Autodesk Inventor part; units mm, degrees
(part 4 of 6)
sketch "Sketch55" plane through (0, 0, 10) normal (0, 0, 1) x (1, 0, 0)
  line L0 (103.1549, -6.3815) -> (106.5137, -3.0228) projected
  line L1 (103.1549, -6.3815) -> (104.357, -7.5836) projected
  line L2 (104.357, -7.5836) -> (100.1144, -11.8263) projected
  line L3 (100.1144, -11.8263) -> (83.8509, -28.0897) projected
  line L4 (83.8509, -28.0897) -> (80.3154, -31.6252) projected
  line L5 (80.3154, -31.6252) -> (71.5473, -22.8571) projected
  line L6 (71.5473, -22.8571) -> (75.0828, -19.3216) projected
  line L7 (75.0828, -19.3216) -> (91.3463, -3.0581) projected
  line L8 (91.3463, -3.0581) -> (95.5889, 1.1845) projected
  line L9 (95.5889, 1.1845) -> (96.791, -0.0176) projected
  line L10 (100.1497, 3.3412) -> (96.791, -0.0176) projected
  line L11 (106.5137, -3.0228) -> (100.1497, 3.3412) projected
  line L12 (4.5, 17.5) -> (4.5, 22.25) projected
  line L13 (4.5, 17.5) -> (6.2, 17.5) projected
  line L14 (6.2, 17.5) -> (6.2, 11.5) projected
  line L15 (6.2, 11.5) -> (6.2, -11.5) projected
  line L16 (6.2, -11.5) -> (6.2, -16.5) projected
  line L17 (6.2, -16.5) -> (-6.2, -16.5) projected
  line L18 (-6.2, -16.5) -> (-6.2, -11.5) projected
  line L19 (-6.2, -11.5) -> (-6.2, 11.5) projected
  line L20 (-6.2, 11.5) -> (-6.2, 17.5) projected
  line L21 (-6.2, 17.5) -> (-4.5, 17.5) projected
  line L22 (-4.5, 22.25) -> (-4.5, 17.5) projected
  line L23 (4.5, 22.25) -> (-4.5, 22.25) projected
  line L24 (-103.1549, -136.2186) -> (-106.5137, -139.5774) projected
  line L25 (-103.1549, -136.2186) -> (-104.357, -135.0165) projected
  line L26 (-104.357, -135.0165) -> (-100.1144, -130.7739) projected
  line L27 (-100.1144, -130.7739) -> (-83.8509, -114.5104) projected
  line L28 (-83.8509, -114.5104) -> (-80.3154, -110.9749) projected
  line L29 (-80.3154, -110.9749) -> (-71.5473, -119.743) projected
  line L30 (-71.5473, -119.743) -> (-75.0828, -123.2786) projected
  line L31 (-75.0828, -123.2786) -> (-91.3463, -139.542) projected
  line L32 (-91.3463, -139.542) -> (-95.5889, -143.7847) projected
  line L33 (-95.5889, -143.7847) -> (-96.791, -142.5826) projected
  line L34 (-100.1497, -145.9413) -> (-96.791, -142.5826) projected
  line L35 (-106.5137, -139.5774) -> (-100.1497, -145.9413) projected
  line L36 (-96.791, -0.0176) -> (-100.1497, 3.3412) projected
  line L37 (-96.791, -0.0176) -> (-95.5889, 1.1845) projected
  line L38 (-95.5889, 1.1845) -> (-91.3463, -3.0581) projected
  line L39 (-91.3463, -3.0581) -> (-75.0828, -19.3216) projected
  line L40 (-75.0828, -19.3216) -> (-71.5473, -22.8571) projected
  line L41 (-71.5473, -22.8571) -> (-80.3154, -31.6252) projected
  line L42 (-80.3154, -31.6252) -> (-83.8509, -28.0897) projected
  line L43 (-83.8509, -28.0897) -> (-100.1144, -11.8263) projected
  line L44 (-100.1144, -11.8263) -> (-104.357, -7.5836) projected
  line L45 (-104.357, -7.5836) -> (-103.1549, -6.3815) projected
  line L46 (-106.5137, -3.0228) -> (-103.1549, -6.3815) projected
  line L47 (-100.1497, 3.3412) -> (-106.5137, -3.0228) projected
  line L48 (-4.5, -160.1002) -> (-4.5, -164.8502) projected
  line L49 (-4.5, -160.1002) -> (-6.2, -160.1002) projected
  line L50 (-6.2, -160.1002) -> (-6.2, -154.1002) projected
  line L51 (-6.2, -154.1002) -> (-6.2, -131.1002) projected
  line L52 (-6.2, -131.1002) -> (-6.2, -126.1002) projected
  line L53 (-6.2, -126.1002) -> (6.2, -126.1002) projected
  line L54 (6.2, -126.1002) -> (6.2, -131.1002) projected
  line L55 (6.2, -131.1002) -> (6.2, -154.1002) projected
  line L56 (6.2, -154.1002) -> (6.2, -160.1002) projected
  line L57 (6.2, -160.1002) -> (4.5, -160.1002) projected
  line L58 (4.5, -164.8502) -> (4.5, -160.1002) projected
  line L59 (-4.5, -164.8502) -> (4.5, -164.8502) projected
  line L60 (96.791, -142.5826) -> (100.1497, -145.9413) projected
  line L61 (96.791, -142.5826) -> (95.5889, -143.7847) projected
  line L62 (95.5889, -143.7847) -> (91.3463, -139.542) projected
  line L63 (91.3463, -139.542) -> (75.0828, -123.2786) projected
  line L64 (75.0828, -123.2786) -> (71.5473, -119.743) projected
  line L65 (71.5473, -119.743) -> (80.3154, -110.9749) projected
  line L66 (80.3154, -110.9749) -> (83.8509, -114.5104) projected
  line L67 (83.8509, -114.5104) -> (100.1144, -130.7739) projected
  line L68 (100.1144, -130.7739) -> (104.357, -135.0165) projected
  line L69 (104.357, -135.0165) -> (103.1549, -136.2186) projected
  line L70 (106.5137, -139.5774) -> (103.1549, -136.2186) projected
  line L71 (100.1497, -145.9413) -> (106.5137, -139.5774) projected
  circle A0 centre (27.1, -49.4001) radius 1.5 projected
  circle A1 centre (-27.1, -49.4001) radius 1.5 projected
  circle A2 centre (27.1, -93.2001) radius 1.5 projected
  circle A3 centre (-27.1, -93.2001) radius 1.5 projected
  line L72 (4.575, -111.1002) -> (4.575, -104.5252) projected
  line L73 (4.575, -104.5252) -> (6.575, -104.5252) projected
  line L74 (6.575, -104.5252) -> (6.575, -111.1002) projected
  line L75 (6.575, -111.1002) -> (4.575, -111.1002) projected
  line L76 (62.0897, -34.6128) -> (57.4405, -39.262) projected
  line L77 (57.4405, -39.262) -> (56.0263, -37.8478) projected
  line L78 (56.0263, -37.8478) -> (60.6755, -33.1986) projected
  line L79 (60.6755, -33.1986) -> (62.0897, -34.6128) projected
  line L80 (-62.0897, -34.6128) -> (-57.4405, -39.262) projected
  line L81 (-62.0897, -34.6128) -> (-60.6755, -33.1986) projected
  line L82 (-60.6755, -33.1986) -> (-56.0263, -37.8478) projected
  line L83 (-56.0263, -37.8478) -> (-57.4405, -39.262) projected
  line L84 (-62.0897, -107.9874) -> (-57.4405, -103.3382) projected
  line L85 (-57.4405, -103.3382) -> (-56.0263, -104.7524) projected
  line L86 (-56.0263, -104.7524) -> (-60.6755, -109.4016) projected
  line L87 (-60.6755, -109.4016) -> (-62.0897, -107.9874) projected
  line L88 (68.5597, -101.5174) -> (63.9105, -96.8681) projected
  line L89 (63.9105, -96.8681) -> (65.3247, -95.4539) projected
  line L90 (65.3247, -95.4539) -> (69.974, -100.1031) projected
  line L91 (69.974, -100.1031) -> (68.5597, -101.5174) projected
  line L92 (84.2822, -48.8001) -> (88.2822, -48.8001) projected
  line L93 (88.2822, -48.8001) -> (94.3529, -27.4901) projected
  line L94 (94.3529, -27.4901) -> (106.8333, -15.0097) projected
  arc A4 (106.8333, -15.0097) -> (88.1629, 3.6608) centre (97.4981, -5.6744) ccw projected
  line L95 (88.1629, 3.6608) -> (75.6824, -8.8196) projected
  line L96 (75.6824, -8.8196) -> (57.202, -21.3001) projected
  line L97 (57.202, -21.3001) -> (38.202, -31.3001) projected
  line L98 (38.202, -31.3001) -> (19.202, -21.3001) projected
  line L99 (19.202, -21.3001) -> (13.202, -3.65) projected
  line L100 (13.202, -3.65) -> (13.202, 14) projected
  arc A5 (13.202, 14) -> (-13.202, 14) centre (0, 14) ccw projected
  line L101 (-13.202, 14) -> (-13.202, -3.65) projected
  line L102 (-13.202, -3.65) -> (-19.202, -21.3001) projected
  line L103 (-19.202, -21.3001) -> (-38.202, -31.3001) projected
  line L104 (-38.202, -31.3001) -> (-57.202, -21.3001) projected
  line L105 (-57.202, -21.3001) -> (-75.6824, -8.8196) projected
  line L106 (-75.6824, -8.8196) -> (-88.1629, 3.6608) projected
  arc A6 (-88.1629, 3.6608) -> (-106.8333, -15.0097) centre (-97.4981, -5.6744) ccw projected
  line L107 (-106.8333, -15.0097) -> (-94.3529, -27.4901) projected
  line L108 (-94.3529, -27.4901) -> (-76.3482, -71.3001) projected
  line L109 (-76.3482, -71.3001) -> (-94.3529, -115.1101) projected
  line L110 (-94.3529, -115.1101) -> (-106.8333, -127.5905) projected
  arc A7 (-106.8333, -127.5905) -> (-88.1629, -146.2609) centre (-97.4981, -136.9257) ccw projected
  line L111 (-88.1629, -146.2609) -> (-75.6824, -133.7805) projected
  line L112 (-75.6824, -133.7805) -> (-57.202, -121.3001) projected
  line L113 (-57.202, -121.3001) -> (-38.202, -111.3001) projected
  line L114 (-38.202, -111.3001) -> (-19.202, -121.3001) projected
  line L115 (-19.202, -121.3001) -> (-13.202, -138.9501) projected
  line L116 (-13.202, -138.9501) -> (-13.202, -156.6002) projected
  arc A8 (-13.202, -156.6002) -> (13.202, -156.6002) centre (0, -156.6002) ccw projected
  line L117 (13.202, -156.6002) -> (13.202, -138.9501) projected
  line L118 (13.202, -138.9501) -> (19.202, -121.3001) projected
  line L119 (19.202, -121.3001) -> (38.202, -111.3001) projected
  line L120 (38.202, -111.3001) -> (57.202, -121.3001) projected
  line L121 (57.202, -121.3001) -> (75.6824, -133.7805) projected
  line L122 (75.6824, -133.7805) -> (88.1629, -146.2609) projected
  arc A9 (88.1629, -146.2609) -> (106.8333, -127.5905) centre (97.4981, -136.9257) ccw projected
  line L123 (106.8333, -127.5905) -> (94.3529, -115.1101) projected
  line L124 (94.3529, -115.1101) -> (88.2822, -93.8001) projected
  line L125 (88.2822, -93.8001) -> (84.2822, -93.8001) projected
  line L126 (84.2822, -48.8001) -> (84.2822, -93.8001) projected
  line L127 (-54.1, -54.2001) -> (44.1, -54.2001) projected
  arc A10 (44.1, -64.2001) -> (44.1, -54.2001) centre (44.1, -59.2001) ccw projected
  line L128 (44.1, -64.2001) -> (44.1, -78.4001) projected
  arc A11 (44.1, -88.4001) -> (44.1, -78.4001) centre (44.1, -83.4001) ccw projected
  line L129 (44.1, -88.4001) -> (-54.1, -88.4001) projected
  line L130 (-54.1, -54.2001) -> (-54.1, -88.4001) projected
  line L131 (-4.575, -38.075) -> (-4.575, -31.5) projected
  line L132 (-4.575, -38.075) -> (-6.575, -38.075) projected
  line L133 (-6.575, -38.075) -> (-6.575, -31.5) projected
  line L134 (-6.575, -31.5) -> (-4.575, -31.5) projected
  line L135 (-4.575, -111.1002) -> (-6.575, -111.1002) projected
  line L136 (-6.575, -111.1002) -> (-6.575, -104.5252) projected
  line L137 (-6.575, -104.5252) -> (-4.575, -104.5252) projected
  line L138 (-4.575, -111.1002) -> (-4.575, -104.5252) projected
  line L139 (4.575, -31.5) -> (6.575, -31.5) projected
  line L140 (6.575, -31.5) -> (6.575, -38.075) projected
  line L141 (6.575, -38.075) -> (4.575, -38.075) projected
  line L142 (4.575, -38.075) -> (4.575, -31.5) projected
  line L143 (68.5597, -41.0828) -> (69.974, -42.497) projected
  line L144 (69.974, -42.497) -> (65.3247, -47.1462) projected
  line L145 (65.3247, -47.1462) -> (63.9105, -45.732) projected
  line L146 (68.5597, -41.0828) -> (63.9105, -45.732) projected
  line L147 (62.0897, -107.9874) -> (60.6755, -109.4016) projected
  line L148 (60.6755, -109.4016) -> (56.0263, -104.7524) projected
  line L149 (56.0263, -104.7524) -> (57.4405, -103.3382) projected
  line L150 (62.0897, -107.9874) -> (57.4405, -103.3382) projected
  line L151 (-68.5597, -101.5174) -> (-69.974, -100.1031) projected
  line L152 (-69.974, -100.1031) -> (-65.3247, -95.4539) projected
  line L153 (-65.3247, -95.4539) -> (-63.9105, -96.8681) projected
  line L154 (-68.5597, -101.5174) -> (-63.9105, -96.8681) projected
  line L155 (-63.9105, -45.732) -> (-65.3247, -47.1462) projected
  line L156 (-65.3247, -47.1462) -> (-69.974, -42.497) projected
  line L157 (-69.974, -42.497) -> (-68.5597, -41.0828) projected
  line L158 (-68.5597, -41.0828) -> (-63.9105, -45.732) projected
  line L159 (106.8333, -15.0097) -> (94.3529, -27.4901) projected
  line L160 (75.6824, -8.8196) -> (94.3529, -27.4901)
  line L161 (94.3529, -115.1101) -> (88.2822, -93.8001) projected
  line L162 (94.3529, -115.1101) -> (75.6824, -133.7805)
  line L163 (13.202, -138.9501) -> (-13.202, -138.9501)
  line L164 (-57.202, -121.3001) -> (-75.6824, -133.7805) projected
  line L165 (-75.6824, -133.7805) -> (-94.3529, -115.1101)
  line L166 (-94.3529, -27.4901) -> (-75.6824, -8.8196)
  line L167 (-19.202, -21.3001) -> (-13.202, -3.65) projected
  line L168 (-13.202, -3.65) -> (13.202, -3.65)
  line L169 (6.2, 11.5) -> (6.2, -11.5) projected
  line L170 (94.3529, -27.4901) -> (88.2822, -48.8001) projected
  line L171 (84.2822, -48.8001) -> (88.2822, -48.8001) projected
  line L172 (94.3529, -27.4901) -> (88.2822, -48.8001)
  line L173 (88.2822, -48.8001) -> (84.4352, -47.7042)
  line L174 (84.4352, -47.7042) -> (90.5059, -26.3942)
  line L175 (90.5059, -26.3942) -> (94.3529, -27.4901)
  line L176 (84.4352, -47.7042) -> (84.2822, -48.8001)
  line L177 (90.5059, -26.3942) -> (91.8815, -25.0187)
  line L178 (88.2822, -93.8001) -> (94.3529, -115.1101)
  line L179 (94.3529, -115.1101) -> (90.5059, -116.206)
  line L180 (90.5059, -116.206) -> (84.4352, -94.896)
  line L181 (84.4352, -94.896) -> (88.2822, -93.8001)
  line L182 (84.2822, -93.8001) -> (84.4352, -94.896)
  line L183 (90.5059, -116.206) -> (91.8815, -117.5815)
  line L184 (75.6824, -8.8196) -> (88.1629, 3.6608) projected
  line L185 (57.202, -21.3001) -> (75.6824, -8.8196) projected
  line L186 (75.6824, -8.8196) -> (57.202, -21.3001)
  line L187 (57.202, -21.3001) -> (59.4406, -24.615)
  line L188 (59.4406, -24.615) -> (77.9211, -12.1345)
  line L189 (77.9211, -12.1345) -> (75.6824, -8.8196)
  line L190 (77.9211, -12.1345) -> (78.4592, -11.5964)
  line L191 (38.202, -31.3001) -> (57.202, -21.3001) projected
  line L192 (38.202, -31.3001) -> (57.202, -21.3001)
  line L193 (57.202, -21.3001) -> (59.065, -24.8397)
  line L194 (59.065, -24.8397) -> (40.065, -34.8397)
  line L195 (40.065, -34.8397) -> (38.202, -31.3001)
  line L196 (59.065, -24.8397) -> (59.4406, -24.615)
  line L197 (19.202, -21.3001) -> (38.202, -31.3001)
  line L198 (38.202, -31.3001) -> (36.339, -34.8397)
  line L199 (36.339, -34.8397) -> (17.339, -24.8397)
  line L200 (17.339, -24.8397) -> (19.202, -21.3001)
  line L201 (36.339, -34.8397) -> (40.065, -34.8397)
  line L202 (13.202, 14) -> (13.202, -3.65) projected
  line L203 (13.202, -3.65) -> (19.202, -21.3001)
  line L204 (19.202, -21.3001) -> (15.4148, -22.5875)
  line L205 (15.4148, -22.5875) -> (9.4148, -4.9375)
  line L206 (9.4148, -4.9375) -> (13.202, -3.65)
  line L207 (15.4148, -22.5875) -> (17.339, -24.8397)
  line L208 (9.4148, -4.9375) -> (9.4148, -3.65)
  line L209 (-13.202, -3.65) -> (-19.202, -21.3001)
  line L210 (-19.202, -21.3001) -> (-15.4148, -22.5875)
  line L211 (-15.4148, -22.5875) -> (-9.4148, -4.9375)
  line L212 (-9.4148, -4.9375) -> (-13.202, -3.65)
  line L213 (-9.4148, -4.9375) -> (-9.4148, -3.65)
  line L214 (-38.202, -31.3001) -> (-19.202, -21.3001) projected
  line L215 (-19.202, -21.3001) -> (-38.202, -31.3001)
  line L216 (-38.202, -31.3001) -> (-36.339, -34.8397)
  line L217 (-36.339, -34.8397) -> (-17.339, -24.8397)
  line L218 (-17.339, -24.8397) -> (-19.202, -21.3001)
  line L219 (-15.4148, -22.5875) -> (-17.339, -24.8397)
  line L220 (-75.6824, -8.8196) -> (-57.202, -21.3001) projected
  line L221 (-38.202, -31.3001) -> (-57.202, -21.3001)
  line L222 (-57.202, -21.3001) -> (-59.065, -24.8397)
  line L223 (-59.065, -24.8397) -> (-40.065, -34.8397)
  line L224 (-40.065, -34.8397) -> (-38.202, -31.3001)
  line L225 (-40.065, -34.8397) -> (-36.339, -34.8397)
  line L226 (-75.6824, -8.8196) -> (-57.202, -21.3001)
  line L227 (-57.202, -21.3001) -> (-59.4406, -24.615)
  line L228 (-59.4406, -24.615) -> (-77.9211, -12.1345)
  line L229 (-77.9211, -12.1345) -> (-75.6824, -8.8196)
  line L230 (-59.4406, -24.615) -> (-59.065, -24.8397)
  line L231 (-77.9211, -12.1345) -> (-78.4592, -11.5964)
  line L232 (-94.3529, -27.4901) -> (-76.3482, -71.3001)
  line L233 (-76.3482, -71.3001) -> (-72.6485, -69.7796)
  line L234 (-72.6485, -69.7796) -> (-90.6531, -25.9696)
  line L235 (-90.6531, -25.9696) -> (-94.3529, -27.4901)
  line L236 (-90.6531, -25.9696) -> (-91.7428, -24.88)
  line L237 (-94.3529, -115.1101) -> (-76.3482, -71.3001) projected
  line L238 (-76.3482, -71.3001) -> (-94.3529, -115.1101)
  line L239 (-94.3529, -115.1101) -> (-90.6531, -116.6306)
  line L240 (-90.6531, -116.6306) -> (-72.6485, -72.8206)
  line L241 (-72.6485, -72.8206) -> (-76.3482, -71.3001)
  line L242 (-72.6485, -69.7796) -> (-72.6485, -72.8206)
  line L243 (-90.6531, -116.6306) -> (-91.7428, -117.7202)
  line L244 (-75.6824, -133.7805) -> (-57.202, -121.3001)
  line L245 (-57.202, -121.3001) -> (-59.4406, -117.9852)
  line L246 (-59.4406, -117.9852) -> (-77.9211, -130.4656)
  line L247 (-77.9211, -130.4656) -> (-75.6824, -133.7805)
  line L248 (-77.9211, -130.4656) -> (-78.4592, -131.0037)
  line L249 (-57.202, -121.3001) -> (-38.202, -111.3001)
  line L250 (-38.202, -111.3001) -> (-40.065, -107.7604)
  line L251 (-40.065, -107.7604) -> (-59.065, -117.7604)
  line L252 (-59.065, -117.7604) -> (-57.202, -121.3001)
  line L253 (-59.065, -117.7604) -> (-59.4406, -117.9852)
  line L254 (-19.202, -121.3001) -> (-38.202, -111.3001) projected
  line L255 (-19.202, -121.3001) -> (-38.202, -111.3001)
  line L256 (-38.202, -111.3001) -> (-36.339, -107.7604)
  line L257 (-36.339, -107.7604) -> (-17.339, -117.7604)
  line L258 (-17.339, -117.7604) -> (-19.202, -121.3001)
  line L259 (-40.065, -107.7604) -> (-36.339, -107.7604)
  line L260 (-13.202, -138.9501) -> (-19.202, -121.3001) projected
  line L261 (-19.202, -121.3001) -> (-13.202, -138.9501)
  line L262 (-13.202, -138.9501) -> (-9.4148, -137.6627)
  line L263 (-9.4148, -137.6627) -> (-15.4148, -120.0127)
  line L264 (-15.4148, -120.0127) -> (-19.202, -121.3001)
  line L265 (-17.339, -117.7604) -> (-15.4148, -120.0127)
  line L266 (-9.4148, -137.6627) -> (-9.4148, -138.9501)
  line L267 (13.202, -138.9501) -> (19.202, -121.3001)
  line L268 (19.202, -121.3001) -> (15.4148, -120.0127)
  line L269 (15.4148, -120.0127) -> (9.4148, -137.6627)
  line L270 (9.4148, -137.6627) -> (13.202, -138.9501)
  line L271 (9.4148, -137.6627) -> (9.4148, -138.9501)
  line L272 (57.202, -121.3001) -> (38.202, -111.3001) projected
  line L273 (19.202, -121.3001) -> (38.202, -111.3001)
  line L274 (38.202, -111.3001) -> (36.339, -107.7604)
  line L275 (36.339, -107.7604) -> (17.339, -117.7604)
  line L276 (17.339, -117.7604) -> (19.202, -121.3001)
  line L277 (17.339, -117.7604) -> (15.4148, -120.0127)
  line L278 (75.6824, -133.7805) -> (57.202, -121.3001) projected
  line L279 (57.202, -121.3001) -> (38.202, -111.3001)
  line L280 (38.202, -111.3001) -> (40.065, -107.7604)
  line L281 (40.065, -107.7604) -> (59.065, -117.7604)
  line L282 (59.065, -117.7604) -> (57.202, -121.3001)
  line L283 (36.339, -107.7604) -> (40.065, -107.7604)
  line L284 (57.202, -121.3001) -> (75.6824, -133.7805)
  line L285 (75.6824, -133.7805) -> (77.9211, -130.4656)
  line L286 (77.9211, -130.4656) -> (59.4406, -117.9852)
  line L287 (59.4406, -117.9852) -> (57.202, -121.3001)
  line L288 (59.065, -117.7604) -> (59.4406, -117.9852)
  line L289 (77.9211, -130.4656) -> (78.4592, -131.0037)
  line L290 (-72.6485, -71.3001) -> (-67.6485, -71.3001)
  line L291 (-67.6485, -71.3001) -> (-67.6485, -56.3001)
  line L292 (-67.6485, -56.3001) -> (-78.1882, -56.3001)
  line L293 (-67.6485, -71.3001) -> (-67.6485, -86.3001)
  line L294 (-67.6485, -71.3001) -> (-52.6485, -71.3001) construction
  line L295 (-67.6485, -86.3001) -> (-78.1882, -86.3001)
  line L296 (84.4352, -94.896) -> (86.627, -102.5899)
  line L297 (86.627, -102.5899) -> (78.9331, -104.7817)
  line L298 (78.9331, -104.7817) -> (76.7413, -97.0878)
  line L299 (76.7413, -97.0878) -> (84.4352, -94.896)
  line L300 (84.4352, -47.7042) -> (86.627, -40.0103)
  line L301 (86.627, -40.0103) -> (78.9331, -37.8185)
  line L302 (78.9331, -37.8185) -> (76.7413, -45.5124)
  line L303 (76.7413, -45.5124) -> (84.4352, -47.7042)
  point P0 (0, 0)
  dimension "d720" = 4
  dimension "d722" = 4
  dimension "d724" = 4
  dimension "d725" = 4
  dimension "d726" = 4
  dimension "d728" = 4
  dimension "d729" = 4
  dimension "d731" = 4
  dimension "d732" = 4
  dimension "d733" = 4
  dimension "d734" = 4
  dimension "d736" = 4
  dimension "d737" = 4
  dimension "d738" = 4
  dimension "d739" = 4
  dimension "d740" = 4
  dimension "d741" = 4
  dimension "d742" = 4
  dimension "d743" = 4
  dimension "d744" = 4
  dimension "d745" = 4
  dimension "d746" = 5
  dimension "d747" = 15
  dimension "d748" = 15
  dimension "d749" = 90
  dimension "d750" = 8
  dimension "d751" = 8
  dimension "d752" = 8
  dimension "d753" = 8
  constraints: 254 end point, 56 equal length, 41 perpendicular, 16 point on line, 3 horizontal, 1 midpoint
  measures "d720" distance of L92.start L92.end
  measures "d722" distance of L92.end L173.end
  measures "d724" distance of L180.end L124.end
  measures "d725" distance of L96.end L187.end
  measures "d726" distance of L194.end L97.end
  measures "d728" distance of L97.end L198.end
  measures "d729" distance of L98.end L204.end
  measures "d731" distance of L102.end L210.end
  measures "d732" distance of L103.end L216.end
  measures "d733" distance of L104.end L222.end
  measures "d734" distance of L104.end L227.end
  measures "d736" distance of L108.end L233.end
  measures "d737" distance of L109.end L239.end
  measures "d738" distance of L112.end L245.end
  measures "d739" distance of L113.end L250.end
  measures "d740" distance of L113.end L256.end
  measures "d741" distance of L263.end L114.end
  measures "d742" distance of L118.end L268.end
  measures "d743" distance of L119.end L274.end
  measures "d744" distance of L119.end L280.end
  measures "d745" distance of L121.end L285.end
  measures "d746" distance of L290.start L290.end
  measures "d747" distance of L290.end L291.end
  measures "d748" distance of L290.end L293.end
  measures "d749" angle of L293 L294
  measures "d750" distance of L180.end L296.end
  measures "d751" distance of L296.end L297.end
  measures "d752" distance of L302.end L173.end
  measures "d753" distance of L300.end L173.end
extrude "Extrusion55" add sketch "Sketch55" along normal up to surface (25 mm away) contours L160 L175 L177 | L190 L189 L160 | L93 L173 L174 L175 | L189 L188 L187 L96 | L92 L176 L173 | L174 L303 L302 L301 | L193 L194 L195 L97 | L187 L196 L193 | L198 L199 L200 L98 | L195 L201 L198 | L125 L181 L182 | L204 L205 L206 L99 | L200 L207 L204 | L124 L179 L180 L181 | L180 L297 L298 L299 | L206 L208 L168 | L162 L183 L179 | L212 L211 L210 L102 | L168 L213 L212 | L285 L289 L162 | L121 L287 L286 L285 | L218 L217 L216 L103 | L210 L219 L218 | L120 L280 L281 L282 | L282 L288 L287 | L224 L223 L222 L104 | L216 L225 L224 | L119 L276 L275 L274 | L274 L283 L280 | L227 L228 L229 L105 | L222 L230 L227 | L118 L270 L269 L268 | L268 L277 L276 | L229 L231 L166 | L163 L271 L270 | L235 L234 L233 L108 | L166 L236 L235 | L262 L266 L163 | L115 L264 L263 L262 | L241 L240 L239 L109 | L233 L242 L241 | L114 L256 L257 L258 | L258 L265 L264 | L239 L243 L165 | L234 L292 L291 L290 L242 | L242 L290 L293 L295 L240 | L113 L252 L251 L250 | L250 L259 L256 | L112 L247 L246 L245 | L245 L253 L252 | L165 L248 L247
sketch "Sketch56" plane through (-78.1882, -86.3001, 35) normal (0, 0, 1) x (1, 0, 0)
  line L0 (0, 0) -> (-12.465, -30.3305) projected
  line L1 (10.5397, 0) -> (0, 0) projected
  line L2 (10.5397, 30) -> (10.5397, 0) projected
  line L3 (0, 30) -> (10.5397, 30) projected
  line L4 (-12.465, 60.3305) -> (0, 30) projected
  line L5 (-13.5546, 61.4201) -> (-12.465, 60.3305) projected
  line L6 (-16.1647, 58.81) -> (-13.5546, 61.4201) projected
  line L7 (1.84, 15) -> (-16.1647, 58.81) projected
  line L8 (-16.1647, -28.81) -> (1.84, 15) projected
  line L9 (-13.5546, -31.4201) -> (-16.1647, -28.81) projected
  line L10 (-12.465, -30.3305) -> (-13.5546, -31.4201) projected
  line L11 (68.7733, 81.3626) -> (62.7733, 63.7126) projected
  line L12 (68.7733, 82.65) -> (68.7733, 81.3626) projected
  line L13 (64.9862, 82.65) -> (68.7733, 82.65) projected
  line L14 (58.9862, 65) -> (64.9862, 82.65) projected
  line L15 (39.9862, 55) -> (58.9862, 65) projected
  line L16 (20.9862, 65) -> (39.9862, 55) projected
  line L17 (2.5057, 77.4804) -> (20.9862, 65) projected
  line L18 (-0.271, 74.7037) -> (2.5057, 77.4804) projected
  line L19 (0.2671, 74.1656) -> (-0.271, 74.7037) projected
  line L20 (18.7475, 61.6851) -> (0.2671, 74.1656) projected
  line L21 (19.1232, 61.4603) -> (18.7475, 61.6851) projected
  line L22 (38.1232, 51.4603) -> (19.1232, 61.4603) projected
  line L23 (41.8491, 51.4603) -> (38.1232, 51.4603) projected
  line L24 (60.8491, 61.4603) -> (41.8491, 51.4603) projected
  line L25 (62.7733, 63.7126) -> (60.8491, 61.4603) projected
  line L26 (95.5272, 61.4603) -> (93.603, 63.7126) projected
  line L27 (114.5272, 51.4603) -> (95.5272, 61.4603) projected
  line L28 (118.2531, 51.4603) -> (114.5272, 51.4603) projected
  line L29 (137.2531, 61.4603) -> (118.2531, 51.4603) projected
  line L30 (137.6288, 61.6851) -> (137.2531, 61.4603) projected
  line L31 (156.1092, 74.1656) -> (137.6288, 61.6851) projected
  line L32 (156.6474, 74.7037) -> (156.1092, 74.1656) projected
  line L33 (153.8706, 77.4804) -> (156.6474, 74.7037) projected
  line L34 (135.3902, 65) -> (153.8706, 77.4804) projected
  line L35 (116.3902, 55) -> (135.3902, 65) projected
  line L36 (97.3902, 65) -> (116.3902, 55) projected
  line L37 (91.3902, 82.65) -> (97.3902, 65) projected
  line L38 (87.603, 82.65) -> (91.3902, 82.65) projected
  line L39 (87.603, 81.3626) -> (87.603, 82.65) projected
  line L40 (93.603, 63.7126) -> (87.603, 81.3626) projected
  line L41 (162.4703, 37.5) -> (162.4703, -7.5) projected
  line L42 (162.6234, -8.5959) -> (162.4703, -7.5) projected
  line L43 (154.9295, -10.7877) -> (162.6234, -8.5959) projected
  line L44 (157.1213, -18.4816) -> (154.9295, -10.7877) projected
  line L45 (164.8152, -16.2898) -> (157.1213, -18.4816) projected
  line L46 (168.6941, -29.9059) -> (164.8152, -16.2898) projected
  line L47 (170.0696, -31.2814) -> (168.6941, -29.9059) projected
  line L48 (172.541, -28.81) -> (170.0696, -31.2814) projected
  line L49 (166.4703, -7.5) -> (172.541, -28.81) projected
  line L50 (166.4703, 37.5) -> (166.4703, -7.5) projected
  line L51 (172.541, 58.81) -> (166.4703, 37.5) projected
  line L52 (170.0696, 61.2814) -> (172.541, 58.81) projected
  line L53 (168.6941, 59.9059) -> (170.0696, 61.2814) projected
  line L54 (164.8152, 46.2898) -> (168.6941, 59.9059) projected
  line L55 (157.1213, 48.4816) -> (164.8152, 46.2898) projected
  line L56 (154.9295, 40.7877) -> (157.1213, 48.4816) projected
  line L57 (162.6234, 38.5959) -> (154.9295, 40.7877) projected
  line L58 (162.4703, 37.5) -> (162.6234, 38.5959) projected
  line L59 (87.603, -51.3626) -> (93.603, -33.7126) projected
  line L60 (87.603, -52.65) -> (87.603, -51.3626) projected
  line L61 (91.3902, -52.65) -> (87.603, -52.65) projected
  line L62 (97.3902, -35) -> (91.3902, -52.65) projected
  line L63 (116.3902, -25) -> (97.3902, -35) projected
  line L64 (135.3902, -35) -> (116.3902, -25) projected
  line L65 (153.8706, -47.4804) -> (135.3902, -35) projected
  line L66 (156.6474, -44.7037) -> (153.8706, -47.4804) projected
  line L67 (156.1092, -44.1656) -> (156.6474, -44.7037) projected
  line L68 (137.6288, -31.6851) -> (156.1092, -44.1656) projected
  line L69 (137.2531, -31.4603) -> (137.6288, -31.6851) projected
  line L70 (118.2531, -21.4603) -> (137.2531, -31.4603) projected
  line L71 (114.5272, -21.4603) -> (118.2531, -21.4603) projected
  line L72 (95.5272, -31.4603) -> (114.5272, -21.4603) projected
  line L73 (93.603, -33.7126) -> (95.5272, -31.4603) projected
  line L74 (39.9862, -25) -> (20.9862, -35) projected
  line L75 (58.9862, -35) -> (39.9862, -25) projected
  line L76 (64.9862, -52.65) -> (58.9862, -35) projected
  line L77 (68.7733, -52.65) -> (64.9862, -52.65) projected
  line L78 (68.7733, -51.3626) -> (68.7733, -52.65) projected
  line L79 (62.7733, -33.7126) -> (68.7733, -51.3626) projected
  line L80 (60.8491, -31.4603) -> (62.7733, -33.7126) projected
  line L81 (41.8491, -21.4603) -> (60.8491, -31.4603) projected
  line L82 (38.1232, -21.4603) -> (41.8491, -21.4603) projected
  line L83 (19.1232, -31.4603) -> (38.1232, -21.4603) projected
  line L84 (18.7475, -31.6851) -> (19.1232, -31.4603) projected
  line L85 (0.2671, -44.1656) -> (18.7475, -31.6851) projected
  line L86 (20.9862, -35) -> (2.5057, -47.4804) projected
  line L87 (-0.271, -44.7037) -> (0.2671, -44.1656) projected
  line L88 (2.5057, -47.4804) -> (-0.271, -44.7037) projected
  point P0 (78.1882, 86.3001)
extrude "Extrusion56" add sketch "Sketch56" along normal blind 20
ref_plane "Work Plane2" through (94.3529, -27.4901, 10) normal (1, 0, 0) x (0, 0, 1)
sketch "Sketch58" plane through (94.3529, -27.4901, 10) normal (1, 0, 0) x (0, 0, 1)
  line L0 (0, -23.8401) -> (45, -23.8401) projected
  line L1 (0, 111.46) -> (45, 111.46) projected
  line L2 (45, -23.8401) -> (45, -22.5526) projected
  arc A0 (45, -23.8401) -> (45, 111.46) centre (-121.8037, 43.81) ccw
  line L3 (45, -23.8401) -> (45, 111.46)
  line L4 (45, 106.2904) -> (45, 93.81) projected
  point P0 (-10, -27.4901)
  dimension "d758" = 180
  constraints: 2 end point, 2 point on circle, 1 centre point, 1 collinear
  measures "d758" radius of A0
extrude "Extrusion57" add sketch "Sketch58" against normal up to surface (188.7058 mm away)
sketch "Sketch61" plane through (94.3529, -27.4901, 55) normal (0, 0, -1) x (-1, 0, 0)
  line L0 (6.0707, -66.31) -> (0, -87.62) projected
  line L1 (0, -87.62) -> (-12.4804, -100.1004) projected
  arc A0 (-12.4804, -100.1004) -> (6.19, -118.7709) centre (-3.1452, -109.4356) ccw projected
  line L2 (6.19, -118.7709) -> (18.6704, -106.2904) projected
  line L3 (18.6704, -106.2904) -> (37.1509, -93.81) projected
  line L4 (37.1509, -93.81) -> (56.1509, -83.81) projected
  line L5 (56.1509, -83.81) -> (75.1509, -93.81) projected
  line L6 (75.1509, -93.81) -> (81.1509, -111.46) projected
  line L7 (81.1509, -111.46) -> (81.1509, -129.1101) projected
  arc A1 (81.1509, -129.1101) -> (107.5549, -129.1101) centre (94.3529, -129.1101) ccw projected
  line L8 (107.5549, -129.1101) -> (107.5549, -111.46) projected
  line L9 (107.5549, -111.46) -> (113.5549, -93.81) projected
  line L10 (113.5549, -93.81) -> (132.5549, -83.81) projected
  line L11 (132.5549, -83.81) -> (151.5549, -93.81) projected
  line L12 (151.5549, -93.81) -> (170.0353, -106.2904) projected
  line L13 (170.0353, -106.2904) -> (182.5158, -118.7709) projected
  arc A2 (182.5158, -118.7709) -> (201.1862, -100.1004) centre (191.851, -109.4356) ccw projected
  line L14 (201.1862, -100.1004) -> (188.7058, -87.62) projected
  line L15 (188.7058, -87.62) -> (170.7011, -43.81) projected
  line L16 (170.7011, -43.81) -> (188.7058, 0) projected
  line L17 (188.7058, 0) -> (201.1862, 12.4804) projected
  arc A3 (201.1862, 12.4804) -> (182.5158, 31.1509) centre (191.851, 21.8157) ccw projected
  line L18 (182.5158, 31.1509) -> (170.0353, 18.6704) projected
  line L19 (170.0353, 18.6704) -> (151.5549, 6.19) projected
  line L20 (151.5549, 6.19) -> (132.5549, -3.81) projected
  line L21 (132.5549, -3.81) -> (113.5549, 6.19) projected
  line L22 (113.5549, 6.19) -> (107.5549, 23.8401) projected
  line L23 (107.5549, 23.8401) -> (107.5549, 41.4901) projected
  arc A4 (107.5549, 41.4901) -> (81.1509, 41.4901) centre (94.3529, 41.4901) ccw projected
  line L24 (81.1509, 41.4901) -> (81.1509, 23.8401) projected
  line L25 (81.1509, 23.8401) -> (75.1509, 6.19) projected
  line L26 (75.1509, 6.19) -> (56.1509, -3.81) projected
  line L27 (56.1509, -3.81) -> (37.1509, 6.19) projected
  line L28 (37.1509, 6.19) -> (18.6704, 18.6704) projected
  line L29 (18.6704, 18.6704) -> (6.19, 31.1509) projected
  arc A5 (6.19, 31.1509) -> (-12.4804, 12.4804) centre (-3.1452, 21.8157) ccw projected
  line L30 (-12.4804, 12.4804) -> (0, 0) projected
  line L31 (0, 0) -> (6.0707, -21.31) projected
  line L32 (6.0707, -66.31) -> (6.0707, -21.31) projected
  line L33 (65.4631, -18.81) -> (69.0427, -18.81) projected
  line L34 (69.0427, -18.81) -> (70.8325, -21.91) projected
  line L35 (70.8325, -21.91) -> (69.0427, -25.01) projected
  line L36 (69.0427, -25.01) -> (65.4631, -25.01) projected
  line L37 (65.4631, -25.01) -> (63.6733, -21.91) projected
  line L38 (63.6733, -21.91) -> (65.4631, -18.81) projected
  line L39 (117.8733, -21.91) -> (119.6631, -18.81) projected
  line L40 (119.6631, -18.81) -> (123.2427, -18.81) projected
  line L41 (123.2427, -18.81) -> (125.0325, -21.91) projected
  line L42 (125.0325, -21.91) -> (123.2427, -25.01) projected
  line L43 (123.2427, -25.01) -> (119.6631, -25.01) projected
  line L44 (119.6631, -25.01) -> (117.8733, -21.91) projected
  line L45 (69.0427, -62.61) -> (70.8325, -65.71) projected
  line L46 (70.8325, -65.71) -> (69.0427, -68.81) projected
  line L47 (69.0427, -68.81) -> (65.4631, -68.81) projected
  line L48 (65.4631, -68.81) -> (63.6733, -65.71) projected
  line L49 (63.6733, -65.71) -> (65.4631, -62.61) projected
  line L50 (65.4631, -62.61) -> (69.0427, -62.61) projected
  line L51 (119.6631, -68.81) -> (117.8733, -65.71) projected
  line L52 (117.8733, -65.71) -> (119.6631, -62.61) projected
  line L53 (119.6631, -62.61) -> (123.2427, -62.61) projected
  line L54 (123.2427, -62.61) -> (125.0325, -65.71) projected
  line L55 (125.0325, -65.71) -> (123.2427, -68.81) projected
  line L56 (123.2427, -68.81) -> (119.6631, -68.81) projected
  line L57 (91.2313, -99.3917) -> (94.3313, -97.6019) projected
  line L58 (94.3313, -97.6019) -> (97.4313, -99.3917) projected
  line L59 (97.4313, -99.3917) -> (97.4313, -102.9713) projected
  line L60 (97.4313, -102.9713) -> (94.3313, -104.7611) projected
  line L61 (94.3313, -104.7611) -> (91.2313, -102.9713) projected
  line L62 (91.2313, -102.9713) -> (91.2313, -99.3917) projected
  line L63 (91.1005, 13.4938) -> (92.7276, 16.3077) projected
  line L64 (92.7276, 16.3077) -> (95.9781, 16.3055) projected
  line L65 (95.9781, 16.3055) -> (97.6015, 13.4894) projected
  line L66 (97.6015, 13.4894) -> (95.9743, 10.6755) projected
  line L67 (95.9743, 10.6755) -> (92.7238, 10.6777) projected
  line L68 (92.7238, 10.6777) -> (91.1005, 13.4938) projected
  line L69 (17.4084, -93.3427) -> (13.8197, -92.2431) projected
  line L70 (13.8197, -92.2431) -> (12.9777, -88.5855) projected
  line L71 (12.9777, -88.5855) -> (15.7243, -86.0274) projected
  line L72 (15.7243, -86.0274) -> (19.313, -87.127) projected
  line L73 (19.313, -87.127) -> (20.155, -90.7847) projected
  line L74 (20.155, -90.7847) -> (17.4084, -93.3427) projected
  line L75 (168.4107, -90.7107) -> (169.2997, -87.0641) projected
  line L76 (169.2997, -87.0641) -> (172.9022, -86.0107) projected
  line L77 (172.9022, -86.0107) -> (175.6157, -88.6039) projected
  line L78 (175.6157, -88.6039) -> (174.7267, -92.2504) projected
  line L79 (174.7267, -92.2504) -> (171.1242, -93.3038) projected
  line L80 (171.1242, -93.3038) -> (168.4107, -90.7107) projected
  line L81 (175.6861, 0.9694) -> (172.9726, -1.6238) projected
  line L82 (172.9726, -1.6238) -> (169.3701, -0.5704) projected
  line L83 (169.3701, -0.5704) -> (168.4811, 3.0762) projected
  line L84 (168.4811, 3.0762) -> (171.1946, 5.6693) projected
  line L85 (171.1946, 5.6693) -> (174.7971, 4.6159) projected
  line L86 (174.7971, 4.6159) -> (175.6861, 0.9694) projected
  line L87 (17.4412, 5.6455) -> (20.1879, 3.0874) projected
  line L88 (20.1879, 3.0874) -> (19.3458, -0.5703) projected
  line L89 (19.3458, -0.5703) -> (15.7571, -1.6699) projected
  line L90 (15.7571, -1.6699) -> (13.0105, 0.8882) projected
  line L91 (13.0105, 0.8882) -> (13.8526, 4.5459) projected
  line L92 (13.8526, 4.5459) -> (17.4412, 5.6455) projected
  circle A6 centre (2.8652, 15.8053) radius 5 projected
  circle A7 centre (94.3529, -120.6101) radius 5 projected
  circle A8 centre (185.8406, 15.8053) radius 5 projected
  circle A9 centre (185.8406, -103.4252) radius 5 projected
  circle A10 centre (2.8652, -103.4252) radius 5 projected
  circle A11 centre (94.3529, 32.9901) radius 5 projected
  line L93 (58.0139, -7.3497) -> (77.0139, 2.6503) projected
  line L94 (54.2879, -7.3497) -> (58.0139, -7.3497) projected
  line L95 (35.2879, 2.6503) -> (54.2879, -7.3497) projected
  line L96 (77.0139, 2.6503) -> (78.938, 4.9026) projected
  line L97 (78.938, 4.9026) -> (84.938, 22.5526) projected
  line L98 (84.938, 22.5526) -> (84.938, 23.8401) projected
  line L99 (84.938, 23.8401) -> (81.1509, 23.8401) projected
  line L100 (18.6704, 18.6704) -> (15.8937, 15.8937) projected
  line L101 (15.8937, 15.8937) -> (16.4318, 15.3556) projected
  line L102 (16.4318, 15.3556) -> (34.9122, 2.8751) projected
  line L103 (158.2634, -18.2419) -> (159.6776, -19.6562) projected
  line L104 (159.6776, -19.6562) -> (164.3268, -15.0069) projected
  line L105 (164.3268, -15.0069) -> (162.9126, -13.5927) projected
  line L106 (162.9126, -13.5927) -> (158.2634, -18.2419) projected
  line L107 (162.9126, -74.0273) -> (164.3268, -72.613) projected
  line L108 (164.3268, -72.613) -> (159.6776, -67.9638) projected
  line L109 (159.6776, -67.9638) -> (158.2634, -69.378) projected
  line L110 (162.9126, -74.0273) -> (158.2634, -69.378) projected
  line L111 (32.2632, -80.4973) -> (33.6774, -81.9115) projected
  line L112 (33.6774, -81.9115) -> (38.3266, -77.2623) projected
  line L113 (38.3266, -77.2623) -> (36.9124, -75.8481) projected
  line L114 (32.2632, -80.4973) -> (36.9124, -75.8481) projected
  line L115 (25.7931, -13.5927) -> (24.3789, -15.0069) projected
  line L116 (24.3789, -15.0069) -> (29.0281, -19.6562) projected
  line L117 (29.0281, -19.6562) -> (30.4424, -18.2419) projected
  line L118 (25.7931, -13.5927) -> (30.4424, -18.2419) projected
  line L119 (89.7779, -4.0099) -> (87.7779, -4.0099) projected
  line L120 (87.7779, -4.0099) -> (87.7779, -10.5849) projected
  line L121 (87.7779, -10.5849) -> (89.7779, -10.5849) projected
  line L122 (89.7779, -10.5849) -> (89.7779, -4.0099) projected
  line L123 (98.9279, -83.6101) -> (100.9279, -83.6101) projected
  line L124 (100.9279, -83.6101) -> (100.9279, -77.0351) projected
  line L125 (100.9279, -77.0351) -> (98.9279, -77.0351) projected
  line L126 (98.9279, -83.6101) -> (98.9279, -77.0351) projected
  line L127 (98.9279, -10.5849) -> (98.9279, -4.0099) projected
  line L128 (98.9279, -10.5849) -> (100.9279, -10.5849) projected
  line L129 (100.9279, -10.5849) -> (100.9279, -4.0099) projected
  line L130 (100.9279, -4.0099) -> (98.9279, -4.0099) projected
  line L131 (148.4529, -26.71) -> (50.2529, -26.71) projected
  arc A12 (50.2529, -26.71) -> (50.2529, -36.71) centre (50.2529, -31.71) ccw projected
  line L132 (50.2529, -36.71) -> (50.2529, -50.91) projected
  arc A13 (50.2529, -50.91) -> (50.2529, -60.91) centre (50.2529, -55.91) ccw projected
  line L133 (50.2529, -60.91) -> (148.4529, -60.91) projected
  line L134 (148.4529, -26.71) -> (148.4529, -60.91) projected
  line L135 (25.7931, -74.0273) -> (30.4424, -69.378) projected
  line L136 (30.4424, -69.378) -> (29.0281, -67.9638) projected
  line L137 (29.0281, -67.9638) -> (24.3789, -72.613) projected
  line L138 (24.3789, -72.613) -> (25.7931, -74.0273) projected
  line L139 (156.4426, -80.4973) -> (151.7934, -75.8481) projected
  line L140 (151.7934, -75.8481) -> (150.3792, -77.2623) projected
  line L141 (150.3792, -77.2623) -> (155.0284, -81.9115) projected
  line L142 (155.0284, -81.9115) -> (156.4426, -80.4973) projected
  line L143 (156.4426, -7.1227) -> (151.7934, -11.7719) projected
  line L144 (156.4426, -7.1227) -> (155.0284, -5.7085) projected
  line L145 (155.0284, -5.7085) -> (150.3792, -10.3577) projected
  line L146 (150.3792, -10.3577) -> (151.7934, -11.7719) projected
  line L147 (32.2632, -7.1227) -> (36.9124, -11.7719) projected
  line L148 (36.9124, -11.7719) -> (38.3266, -10.3577) projected
  line L149 (38.3266, -10.3577) -> (33.6774, -5.7085) projected
  line L150 (33.6774, -5.7085) -> (32.2632, -7.1227) projected
  line L151 (89.7779, -83.6101) -> (89.7779, -77.0351) projected
  line L152 (89.7779, -77.0351) -> (87.7779, -77.0351) projected
  line L153 (87.7779, -77.0351) -> (87.7779, -83.6101) projected
  line L154 (87.7779, -83.6101) -> (89.7779, -83.6101) projected
  circle A14 centre (121.4529, -65.71) radius 1.5 projected
  circle A15 centre (67.2529, -65.71) radius 1.5 projected
  circle A16 centre (121.4529, -21.91) radius 1.5 projected
  circle A17 centre (67.2529, -21.91) radius 1.5 projected
  line L155 (-2.4381, -115.0925) -> (-5.7969, -118.4512) projected
  line L156 (-2.4381, -115.0925) -> (-1.236, -116.2946) projected
  line L157 (-1.236, -116.2946) -> (3.0066, -112.0519) projected
  line L158 (3.0066, -112.0519) -> (19.2701, -95.7885) projected
  line L159 (19.2701, -95.7885) -> (22.8056, -92.2529) projected
  line L160 (22.8056, -92.2529) -> (14.0375, -83.4848) projected
  line L161 (14.0375, -83.4848) -> (10.5019, -87.0203) projected
  line L162 (10.5019, -87.0203) -> (-5.7615, -103.2838) projected
  line L163 (-5.7615, -103.2838) -> (-10.0041, -107.5264) projected
  line L164 (-10.0041, -107.5264) -> (-8.8021, -108.7285) projected
  line L165 (-12.1608, -112.0873) -> (-8.8021, -108.7285) projected
  line L166 (-5.7969, -118.4512) -> (-12.1608, -112.0873) projected
  line L167 (98.8529, -132.6101) -> (98.8529, -137.3601) projected
  line L168 (98.8529, -132.6101) -> (100.5529, -132.6101) projected
  line L169 (100.5529, -132.6101) -> (100.5529, -126.6101) projected
  line L170 (100.5529, -126.6101) -> (100.5529, -103.6101) projected
  line L171 (100.5529, -103.6101) -> (100.5529, -98.6101) projected
  line L172 (100.5529, -98.6101) -> (88.1529, -98.6101) projected
  line L173 (88.1529, -98.6101) -> (88.1529, -103.6101) projected
  line L174 (88.1529, -103.6101) -> (88.1529, -126.6101) projected
  line L175 (88.1529, -126.6101) -> (88.1529, -132.6101) projected
  line L176 (88.1529, -132.6101) -> (89.8529, -132.6101) projected
  line L177 (89.8529, -137.3601) -> (89.8529, -132.6101) projected
  line L178 (98.8529, -137.3601) -> (89.8529, -137.3601) projected
  line L179 (191.1439, 27.4725) -> (194.5026, 30.8313) projected
  line L180 (191.1439, 27.4725) -> (189.9418, 28.6746) projected
  line L181 (189.9418, 28.6746) -> (185.6991, 24.432) projected
  line L182 (185.6991, 24.432) -> (169.4357, 8.1685) projected
  line L183 (169.4357, 8.1685) -> (165.9002, 4.633) projected
  line L184 (165.9002, 4.633) -> (174.6683, -4.1352) projected
  line L185 (174.6683, -4.1352) -> (178.2038, -0.5996) projected
  line L186 (178.2038, -0.5996) -> (194.4673, 15.6638) projected
  line L187 (194.4673, 15.6638) -> (198.7099, 19.9065) projected
  line L188 (198.7099, 19.9065) -> (197.5078, 21.1086) projected
  line L189 (200.8666, 24.4673) -> (197.5078, 21.1086) projected
  line L190 (194.5026, 30.8313) -> (200.8666, 24.4673) projected
  line L191 (197.5078, -108.7285) -> (200.8666, -112.0873) projected
  line L192 (197.5078, -108.7285) -> (198.7099, -107.5264) projected
  line L193 (198.7099, -107.5264) -> (194.4673, -103.2838) projected
  line L194 (194.4673, -103.2838) -> (178.2038, -87.0203) projected
  line L195 (178.2038, -87.0203) -> (174.6683, -83.4848) projected
  line L196 (174.6683, -83.4848) -> (165.9002, -92.2529) projected
  line L197 (165.9002, -92.2529) -> (169.4357, -95.7885) projected
  line L198 (169.4357, -95.7885) -> (185.6991, -112.0519) projected
  line L199 (185.6991, -112.0519) -> (189.9418, -116.2946) projected
  line L200 (189.9418, -116.2946) -> (191.1439, -115.0925) projected
  line L201 (194.5026, -118.4512) -> (191.1439, -115.0925) projected
  line L202 (200.8666, -112.0873) -> (194.5026, -118.4512) projected
  line L203 (89.8529, 44.9901) -> (89.8529, 49.7401) projected
  line L204 (89.8529, 44.9901) -> (88.1529, 44.9901) projected
  line L205 (88.1529, 44.9901) -> (88.1529, 38.9901) projected
  line L206 (88.1529, 38.9901) -> (88.1529, 15.9901) projected
  line L207 (88.1529, 15.9901) -> (88.1529, 10.9901) projected
  line L208 (88.1529, 10.9901) -> (100.5529, 10.9901) projected
  line L209 (100.5529, 10.9901) -> (100.5529, 15.9901) projected
  line L210 (100.5529, 15.9901) -> (100.5529, 38.9901) projected
  line L211 (100.5529, 38.9901) -> (100.5529, 44.9901) projected
  line L212 (100.5529, 44.9901) -> (98.8529, 44.9901) projected
  line L213 (98.8529, 49.7401) -> (98.8529, 44.9901) projected
  line L214 (89.8529, 49.7401) -> (98.8529, 49.7401) projected
  line L215 (-8.8021, 21.1086) -> (-12.1608, 24.4673) projected
  line L216 (-8.8021, 21.1086) -> (-10.0041, 19.9065) projected
  line L217 (-10.0041, 19.9065) -> (-5.7615, 15.6638) projected
  line L218 (-5.7615, 15.6638) -> (10.5019, -0.5996) projected
  line L219 (10.5019, -0.5996) -> (14.0375, -4.1352) projected
  line L220 (14.0375, -4.1352) -> (22.8056, 4.633) projected
  line L221 (22.8056, 4.633) -> (19.2701, 8.1685) projected
  line L222 (19.2701, 8.1685) -> (3.0066, 24.432) projected
  line L223 (3.0066, 24.432) -> (-1.236, 28.6746) projected
  line L224 (-1.236, 28.6746) -> (-2.4381, 27.4725) projected
  line L225 (-5.7969, 30.8313) -> (-2.4381, 27.4725) projected
  line L226 (-12.1608, 24.4673) -> (-5.7969, 30.8313) projected
  line L227 (107.5549, 23.8401) -> (103.7677, 23.8401) projected
  line L228 (103.7677, 23.8401) -> (103.7677, 22.5526) projected
  line L229 (103.7677, 22.5526) -> (109.7677, 4.9026) projected
  line L230 (109.7677, 4.9026) -> (111.6919, 2.6503) projected
  line L231 (111.6919, 2.6503) -> (130.6919, -7.3497) projected
  line L232 (130.6919, -7.3497) -> (134.4179, -7.3497) projected
  line L233 (134.4179, -7.3497) -> (153.4179, 2.6503) projected
  line L234 (153.4179, 2.6503) -> (153.7935, 2.8751) projected
  line L235 (153.7935, 2.8751) -> (172.274, 15.3556) projected
  line L236 (172.274, 15.3556) -> (172.8121, 15.8937) projected
  line L237 (172.8121, 15.8937) -> (170.0353, 18.6704) projected
  line L238 (170.0353, 18.6704) -> (182.5158, 31.1509) projected
  arc A18 (201.1862, 12.4804) -> (182.5158, 31.1509) centre (191.851, 21.8157) ccw projected
  line L239 (201.1862, 12.4804) -> (188.7058, 0) projected
  line L240 (188.7058, 0) -> (186.0956, 2.6101) projected
  line L241 (186.0956, 2.6101) -> (185.006, 1.5205) projected
  line L242 (185.006, 1.5205) -> (172.541, -28.81) projected
  line L243 (172.541, -28.81) -> (162.0013, -28.81) projected
  line L244 (162.0013, -28.81) -> (162.0013, -58.81) projected
  line L245 (162.0013, -58.81) -> (172.541, -58.81) projected
  line L246 (172.541, -58.81) -> (185.006, -89.1405) projected
  line L247 (185.006, -89.1405) -> (186.0956, -90.2301) projected
  line L248 (186.0956, -90.2301) -> (188.7058, -87.62) projected
  line L249 (188.7058, -87.62) -> (201.1862, -100.1004) projected
  arc A19 (182.5158, -118.7709) -> (201.1862, -100.1004) centre (191.851, -109.4356) ccw projected
  line L250 (182.5158, -118.7709) -> (170.0353, -106.2904) projected
  line L251 (172.274, -102.9755) -> (153.7935, -90.4951) projected
  line L252 (153.7935, -90.4951) -> (153.4179, -90.2703) projected
  line L253 (153.4179, -90.2703) -> (134.4179, -80.2703) projected
  line L254 (134.4179, -80.2703) -> (130.6919, -80.2703) projected
  line L255 (130.6919, -80.2703) -> (111.6919, -90.2703) projected
  line L256 (111.6919, -90.2703) -> (109.7677, -92.5226) projected
  line L257 (109.7677, -92.5226) -> (103.7677, -110.1726) projected
  line L258 (103.7677, -110.1726) -> (103.7677, -111.46) projected
  line L259 (103.7677, -111.46) -> (107.5549, -111.46) projected
  line L260 (107.5549, -111.46) -> (107.5549, -129.1101) projected
  arc A20 (81.1509, -129.1101) -> (107.5549, -129.1101) centre (94.3529, -129.1101) ccw projected
  line L261 (81.1509, -129.1101) -> (81.1509, -111.46) projected
  line L262 (81.1509, -111.46) -> (84.938, -111.46) projected
  line L263 (84.938, -111.46) -> (84.938, -110.1726) projected
  line L264 (84.938, -110.1726) -> (78.938, -92.5226) projected
  line L265 (78.938, -92.5226) -> (77.0139, -90.2703) projected
  line L266 (77.0139, -90.2703) -> (58.0139, -80.2703) projected
  line L267 (58.0139, -80.2703) -> (54.2879, -80.2703) projected
  line L268 (54.2879, -80.2703) -> (35.2879, -90.2703) projected
  line L269 (35.2879, -90.2703) -> (34.9122, -90.4951) projected
  line L270 (34.9122, -90.4951) -> (16.4318, -102.9755) projected
  line L271 (16.4318, -102.9755) -> (15.8937, -103.5137) projected
  line L272 (15.8937, -103.5137) -> (18.6704, -106.2904) projected
  line L273 (18.6704, -106.2904) -> (6.19, -118.7709) projected
  arc A21 (-12.4804, -100.1004) -> (6.19, -118.7709) centre (-3.1452, -109.4356) ccw projected
  line L274 (-12.4804, -100.1004) -> (0, -87.62) projected
  line L275 (0, -87.62) -> (2.4714, -90.0914) projected
  line L276 (2.4714, -90.0914) -> (3.8469, -88.7159) projected
  line L277 (3.8469, -88.7159) -> (7.7259, -75.0998) projected
  line L278 (7.7259, -75.0998) -> (15.4197, -77.2916) projected
  line L279 (15.4197, -77.2916) -> (17.6116, -69.5977) projected
  line L280 (17.6116, -69.5977) -> (9.9177, -67.4059) projected
  line L281 (9.9177, -67.4059) -> (10.0707, -66.31) projected
  line L282 (10.0707, -21.31) -> (10.0707, -66.31) projected
  line L283 (10.0707, -21.31) -> (9.9177, -20.2141) projected
  line L284 (9.9177, -20.2141) -> (17.6116, -18.0223) projected
  line L285 (17.6116, -18.0223) -> (15.4197, -10.3284) projected
  line L286 (15.4197, -10.3284) -> (7.7259, -12.5202) projected
  line L287 (7.7259, -12.5202) -> (3.8469, 1.0959) projected
  line L288 (3.8469, 1.0959) -> (2.4714, 2.4714) projected
  line L289 (2.4714, 2.4714) -> (0, 0) projected
  line L290 (0, 0) -> (-12.4804, 12.4804) projected
  arc A22 (6.19, 31.1509) -> (-12.4804, 12.4804) centre (-3.1452, 21.8157) ccw projected
  line L291 (6.19, 31.1509) -> (18.6704, 18.6704) projected
  line L292 (18.6704, 18.6704) -> (15.8937, 15.8937) projected
  line L293 (15.8937, 15.8937) -> (16.4318, 15.3556) projected
  line L294 (16.4318, 15.3556) -> (34.9122, 2.8751) projected
  line L295 (34.9122, 2.8751) -> (35.2879, 2.6503) projected
  line L296 (35.2879, 2.6503) -> (54.2879, -7.3497) projected
  line L297 (54.2879, -7.3497) -> (58.0139, -7.3497) projected
  line L298 (58.0139, -7.3497) -> (77.0139, 2.6503) projected
  line L299 (77.0139, 2.6503) -> (78.938, 4.9026) projected
  line L300 (78.938, 4.9026) -> (84.938, 22.5526) projected
  line L301 (84.938, 22.5526) -> (84.938, 23.8401) projected
  line L302 (84.938, 23.8401) -> (81.1509, 23.8401) projected
  line L303 (81.1509, 23.8401) -> (81.1509, 41.4901) projected
  arc A23 (107.5549, 41.4901) -> (81.1509, 41.4901) centre (94.3529, 41.4901) ccw projected
  line L304 (107.5549, 41.4901) -> (107.5549, 23.8401) projected
  line L305 (188.7058, 0) -> (186.0956, 2.6101) projected
  line L306 (186.0956, 2.6101) -> (172.8121, 15.8937)
  line L307 (103.7677, 23.8401) -> (103.7677, 22.5526) projected
  line L308 (103.7677, 23.8401) -> (84.938, 23.8401)
  line L309 (88.1529, 38.9901) -> (88.1529, 15.9901) projected
  line L310 (15.8937, 15.8937) -> (2.4714, 2.4714)
  line L311 (15.8937, -103.5137) -> (18.6704, -106.2904) projected
  line L312 (2.4714, -90.0914) -> (15.8937, -103.5137)
  line L313 (84.938, -111.46) -> (84.938, -110.1726) projected
  line L314 (84.938, -111.46) -> (103.7677, -111.46)
  line L315 (172.274, -102.9755) -> (153.7935, -90.4951) projected
  line L316 (186.0956, -90.2301) -> (188.7058, -87.62) projected
  line L317 (175.2049, 23.8401) -> (107.5549, 23.8401)
  line L318 (81.1509, 23.8401) -> (13.5008, 23.8401)
  line L319 (0, 0) -> (0, -87.62)
  line L320 (0, 23.8401) -> (0, -111.46) projected
  line L321 (13.5008, -111.46) -> (81.1509, -111.46)
  line L322 (107.5549, -111.46) -> (175.2049, -111.46)
  line L323 (188.7058, -87.62) -> (188.7058, 0)
  line L324 (188.7058, -111.46) -> (188.7058, 23.8401) projected
  line L325 (170.0353, -106.2904) -> (172.8121, -103.5137) projected
  line L326 (172.8121, -103.5137) -> (172.274, -102.9755) projected
  line L327 (172.8121, -103.5137) -> (186.0956, -90.2301)
  point P0 (94.3529, 27.4901)
  point P1 (15.8937, 15.8937)
  point P2 (13.5008, 23.8401)
  point P3 (0, 0)
  point P4 (0, 0)
  point P5 (0, 0)
  point P6 (0, 0)
  point P7 (13.5008, -111.46)
  point P8 (107.5549, -111.46)
  point P9 (175.2049, -111.46)
  point P10 (175.2049, 23.8401)
  point P11 (170.0353, 18.6704)
  constraints: 24 end point, 6 point on line, 5 perpendicular, 3 collinear, 1 horizontal
extrude "Extrusion58" cut sketch "Sketch61" against normal blind 208.25 contours L0 L319 L31 L32 | L320 L162 L163 L164 L165 L166 L155 L156 L157 L158 L312 L272 L2 A0 L1 | L275 L312 L162 L320 | L320 L218 L310 L289 | L30 A5 L29 L100 L310 L222 L223 L224 L225 L226 L215 L216 L217 L218 L320 | L162 L312 L158 L157 L156 L155 L166 L165 L164 L163 | L218 L217 L216 L215 L226 L225 L224 L223 L222 L310 | L2 L3 L4 L5 L6 L321 | L318 L25 L26 L27 L28 L29 | L9 L10 L11 L12 L13 L322 | L13 L325 L327 L198 L199 L200 L201 L202 L191 L192 L193 L194 L324 L14 A2 | L317 L18 L19 L20 L21 L22 | L18 A3 L17 L324 L186 L187 L188 L189 L190 L179 L180 L181 L182 L306 L237 | L327 L194 L193 L192 L191 L202 L201 L200 L199 L198 | L324 L194 L327 L248 | L15 L16 L323 | L240 L306 L186 L324 | L182 L181 L180 L179 L190 L189 L188 L187 L186 L306 | A6 L320 | L320 A6 | A8 L324 | L324 A8 | A9 L324 | L324 A9 | A10 L320 | L320 A10
sketch "Sketch62" plane through (88.2822, -48.8001, 10) normal (1, 0, 0) x (0, 0, -1)
  line L0 (-6.15, -26.05) -> (-6.15, -19.05) projected
  arc A0 (-2.35, -19.05) -> (-6.15, -19.05) centre (-4.25, -19.05) ccw projected
  line L1 (-2.35, -19.05) -> (-2.35, -26.05) projected
  arc A1 (-6.15, -26.05) -> (-2.35, -26.05) centre (-4.25, -26.05) ccw projected
  line L2 (15, -45) -> (-56.7845, -45) projected
  line L3 (15, -45) -> (15, 0) projected
  line L4 (-56.7845, 0) -> (15, 0) projected
  arc A2 (-56.7845, 0) -> (-56.7845, -45) centre (121.8037, -22.5) ccw projected
  circle A3 centre (-3.5, -1.55) radius 1 projected
  circle A4 centre (-12, -9.05) radius 8.15 projected
  circle A5 centre (-20.5, -1.55) radius 1 projected
  circle A6 centre (-20.5, -43.55) radius 1 projected
  circle A7 centre (-12, -36.05) radius 8.15 projected
  circle A8 centre (-3.5, -43.55) radius 1 projected
  line L5 (-45, -45) -> (0, -45) projected
  line L6 (-56.7845, 0) -> (15, 0) projected
  line L7 (0, -45) -> (0, 0)
  line L8 (0, 0) -> (15, 0)
  line L9 (15, 0) -> (15, -45)
  line L10 (15, -45) -> (0, -45)
  line L11 (0, 0) -> (0, -45) projected
  line L12 (0, 0) -> (0, 84)
  line L13 (0, 84) -> (15, 84)
  line L14 (15, 84) -> (15, 0)
  line L15 (15, 0) -> (0, 0)
  line L16 (0, -45) -> (0, -129)
  line L17 (0, -129) -> (15, -129)
  line L18 (15, -129) -> (15, -45)
  line L19 (15, -45) -> (0, -45)
  point P0 (10, 48.8001)
  dimension "d763" = 0
  dimension "d764" = 0
  dimension "d765" = 84
  dimension "d766" = 0
  dimension "d767" = 129
  constraints: 24 end point, 6 parallel, 4 perpendicular, 3 point on line
  measures "d763" distance between parallel lines of L3 L14
  measures "d764" distance between parallel lines of L3 L9
  measures "d765" distance between parallel lines of L2 L17
  measures "d766" distance between parallel lines of L3 L18
  measures "d767" distance between parallel lines of L5 L13
extrude "Extrusion59" cut sketch "Sketch62" along normal mid plane 529.75 contours L18 L17 L16 L2 | L2 L7 L4 L3 | L4 L12 L13 L14